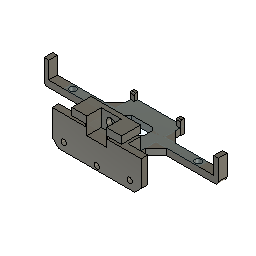
mount v12 (Autodesk Fusion 360 design; units mm, degrees)
Autodesk Fusion 360 part; units mm, degrees
sketch "Sketch1" plane through (0, 0, 0) normal (0, 0, 1) x (1, 0, 0)
  line L0 (51.0982, 3.3166) -> (-51.0982, 3.3166)
  line L1 (-51.0982, 3.3166) -> (-51.0982, -3.3166)
  line L2 (-51.0982, -3.3166) -> (51.0982, -3.3166)
  line L3 (51.0982, -3.3166) -> (51.0982, 3.3166)
  line L4 (51.0982, 3.3166) -> (-51.0982, -3.3166) construction
  line L5 (-51.0982, 3.3166) -> (51.0982, -3.3166) construction
  line L6 (18.7789, 17.5) -> (-18.7789, 17.5)
  line L7 (-18.7789, 17.5) -> (-18.7789, -17.5)
  line L8 (-18.7789, -17.5) -> (18.7789, -17.5)
  line L9 (18.7789, -17.5) -> (18.7789, 17.5)
  line L10 (18.7789, 17.5) -> (-18.7789, -17.5) construction
  line L11 (-18.7789, 17.5) -> (18.7789, -17.5) construction
  dimension "d5" = 35
  constraint horizontal L0
  constraint perpendicular L0 L1
  constraint parallel L0 L2
  constraint parallel L1 L3
  constraint coincident L4 origin
  constraint coincident L5 origin
  constraint horizontal L6
  constraint perpendicular L6 L7
  constraint parallel L6 L8
  constraint parallel L7 L9
  constraint coincident L10 origin
  constraint coincident L11 origin
  measures "d5" distance of L6.start L8.end
extrude "Extrude1" add sketch "Sketch1" along normal blind 5
move_body "Move1" bodies 1 to x (1, 0, 0) y (0, 1, 0) z (0, 0, 1) at (0, 0, -31)
sketch "Sketch2" plane through (0, 0, -31) normal (0, 0, -1) x (1, 0, 0)
  line L0 (18.7789, 3.3166) -> (18.7789, 17.5)
  line L1 (18.7789, 17.5) -> (-18.7789, 17.5)
  line L2 (-18.7789, 17.5) -> (-18.7789, 3.3166)
  line L3 (-18.7789, 3.3166) -> (-51.0982, 3.3166)
  line L4 (-51.0982, 3.3166) -> (-51.0982, -3.3166)
  line L5 (-51.0982, -3.3166) -> (-18.7789, -3.3166)
  line L6 (-18.7789, -3.3166) -> (-18.7789, -17.5)
  line L7 (-18.7789, -17.5) -> (18.7789, -17.5)
  line L8 (18.7789, -17.5) -> (18.7789, -3.3166)
  line L9 (18.7789, -3.3166) -> (51.0982, -3.3166)
  line L10 (51.0982, -3.3166) -> (51.0982, 3.3166)
  line L11 (51.0982, 3.3166) -> (18.7789, 3.3166)
  circle A0 centre (47.5, 0) radius 2.4207
  circle A1 centre (-47.5, 0) radius 2.3964
extrude "Extrude2" cut sketch "Sketch2" against normal blind 5 contours A0 | A1
sketch "Sketch3" plane through (0, 0, -26) normal (0, 0, 1) x (-1, 0, 0)
  circle A0 centre (-47.5, 0) radius 2.4207
  circle A1 centre (47.5, 0) radius 2.3964
  line L0 (-18.7789, 17.5) -> (-18.7789, 3.3166)
  line L1 (-18.7789, 3.3166) -> (-51.0982, 3.3166)
  line L2 (-51.0982, 3.3166) -> (-51.0982, -3.3166)
  line L3 (-51.0982, -3.3166) -> (-18.7789, -3.3166)
  line L4 (-18.7789, -3.3166) -> (-18.7789, -17.5)
  line L5 (-18.7789, -17.5) -> (18.7789, -17.5)
  line L6 (18.7789, -17.5) -> (18.7789, -3.3166)
  line L7 (18.7789, -3.3166) -> (51.0982, -3.3166)
  line L8 (51.0982, -3.3166) -> (51.0982, 3.3166)
  line L9 (51.0982, 3.3166) -> (18.7789, 3.3166)
  line L10 (18.7789, 3.3166) -> (18.7789, 17.5)
  line L11 (18.7789, 17.5) -> (-18.7789, 17.5)
extrude "Extrude3" add 1 faces at (-6.2596, -17.5, -27.6667) along direction (0, -1, 0) blind 12
sketch "Sketch4" plane through (0, 0, -26) normal (0, 0, 1) x (-1, 0, 0)
  circle A0 centre (-47.5, 0) radius 2.4207
  circle A1 centre (47.5, 0) radius 2.3964
  line L0 (-18.7789, 29.5) -> (-18.7789, 3.3166)
  line L1 (-18.7789, 3.3166) -> (-51.0982, 3.3166)
  line L2 (-51.0982, 3.3166) -> (-51.0982, -3.3166)
  line L3 (-51.0982, -3.3166) -> (-18.7789, -3.3166)
  line L4 (-18.7789, -3.3166) -> (-18.7789, -17.5)
  line L5 (-18.7789, -17.5) -> (18.7789, -17.5)
  line L6 (18.7789, -17.5) -> (18.7789, -3.3166)
  line L7 (18.7789, -3.3166) -> (51.0982, -3.3166)
  line L8 (51.0982, -3.3166) -> (51.0982, 3.3166)
  line L9 (51.0982, 3.3166) -> (18.7789, 3.3166)
  line L10 (18.7789, 3.3166) -> (18.7789, 29.5)
  line L11 (18.7789, 29.5) -> (-18.7789, 29.5)
  line L12 (18.7789, 29.5) -> (-18.7789, 29.5)
  line L13 (-18.7789, 29.5) -> (-18.7789, 15.0044)
  line L14 (-18.7789, 15.0044) -> (18.7789, 15.0044)
  line L15 (18.7789, 15.0044) -> (18.7789, 29.5)
  constraint horizontal L12
  constraint vertical L13
  constraint horizontal L14
  constraint vertical L15
  constraint coincident L0 L13.end
  constraint coincident L10.end L11.start
extrude "Extrude4" add sketch "Sketch4" along normal blind 17 contours L0 L10 L11 L12 L13 L14 L15
sketch "Sketch5" plane through (0, -29.5, 0) normal (0, -1, 0) x (1, 0, 0)
  line L0 (-18.7789, -31) -> (18.7789, -31)
  line L1 (18.7789, -31) -> (18.7789, -9)
  line L2 (18.7789, -9) -> (-18.7789, -9)
  line L3 (-18.7789, -9) -> (-18.7789, -31)
  line L4 (-7.4893, -9) -> (7.5, -9)
  line L5 (7.5, -9) -> (7.5, -22)
  line L6 (7.5, -22) -> (-7.4893, -22)
  line L7 (-7.4893, -22) -> (-7.4893, -9)
  constraint horizontal L4
  constraint vertical L5
  constraint horizontal L6
  constraint vertical L7
  constraint coincident L2 L4.start
extrude "Extrude5" cut sketch "Sketch5" against normal blind 11 contours L2 L4 L5 L6 L7
sketch "Sketch6" plane through (0, -29.5, 0) normal (0, -1, 0) x (1, 0, 0)
  line L0 (-7.4893, -22) -> (-7.4893, -9)
  line L1 (-7.4893, -9) -> (-18.7789, -9)
  line L2 (-18.7789, -9) -> (-18.7789, -31)
  line L3 (-18.7789, -31) -> (18.7789, -31)
  line L4 (18.7789, -31) -> (18.7789, -9)
  line L5 (18.7789, -9) -> (7.5, -9)
  line L6 (7.5, -9) -> (7.5, -22)
  line L7 (7.5, -22) -> (-7.4893, -22)
  line L8 (-18.7789, -14.4743) -> (-8.5, -14.4743)
  line L9 (-8.5, -14.4743) -> (-8.5, -16.5)
  line L10 (-8.5, -16.5) -> (-18.7789, -16.5)
  line L11 (-18.7789, -16.5) -> (-18.7789, -14.4743)
  line L12 (18.7789, -14.4808) -> (8.5, -14.4808)
  line L13 (8.5, -14.4808) -> (8.5, -16.5)
  line L14 (8.5, -16.5) -> (18.7789, -16.5)
  line L15 (18.7789, -16.5) -> (18.7789, -14.4808)
  constraint horizontal L8
  constraint vertical L9
  constraint horizontal L10
  constraint vertical L11
  constraint coincident L2 L8.start
  constraint horizontal L12
  constraint vertical L13
  constraint horizontal L14
  constraint vertical L15
  constraint coincident L4 L12.start
extrude "Extrude6" cut sketch "Sketch6" against normal blind 18 contours L2 L8 L9 L10 L11 | L4 L12 L13 L14 L15
sketch "Sketch7" plane through (-18.7789, 0, 0) normal (-1, 0, 0) x (0, -1, 0)
  line L0 (29.5, -16.5) -> (15.0044, -16.5)
  line L1 (15.0044, -16.5) -> (15.0044, -26)
  line L2 (15.0044, -26) -> (3.3166, -26)
  line L3 (3.3166, -26) -> (3.3166, -31)
  line L4 (3.3166, -31) -> (29.5, -31)
  line L5 (29.5, -31) -> (29.5, -16.5)
  line L6 (29.5, -31) -> (24.5, -31)
  line L7 (24.5, -31) -> (24.5, -16.5)
  line L8 (24.5, -16.5) -> (29.5, -16.5)
  line L9 (29.5, -16.5) -> (29.5, -31)
  dimension "d14" = 5
  constraint horizontal L6
  constraint vertical L7
  constraint horizontal L8
  constraint vertical L9
  constraint coincident L4.end L5.start
  measures "d14" distance of L4.end L6.end
sketch "Sketch8" plane through (18.7789, 0, 0) normal (1, 0, 0) x (0, 1, 0)
  line L0 (-15.0044, -16.5) -> (-29.5, -16.5)
  line L1 (-29.5, -16.5) -> (-29.5, -31)
  line L2 (-29.5, -31) -> (-3.3166, -31)
  line L3 (-3.3166, -31) -> (-3.3166, -26)
  line L4 (-3.3166, -26) -> (-15.0044, -26)
  line L5 (-15.0044, -26) -> (-15.0044, -16.5)
  line L6 (-29.5, -31) -> (-24.5, -31)
  line L7 (-24.5, -31) -> (-24.5, -16.5)
  line L8 (-24.5, -16.5) -> (-29.5, -16.5)
  line L9 (-29.5, -16.5) -> (-29.5, -31)
  dimension "d15" = 5
  constraint horizontal L6
  constraint vertical L7
  constraint horizontal L8
  constraint vertical L9
  constraint coincident L1.end L2.start
  measures "d15" distance of L1.end L6.end
extrude "Extrude7" add sketch "Sketch7" along normal blind 15 contours L0 L4 L5 L6 L7 L8 L9
extrude "Extrude8" add sketch "Sketch8" along normal blind 15 contours L0 L1 L2 L6 L7 L8 L9
sketch "Sketch9" plane through (0, 0, -31) normal (0, 0, -1) x (1, 0, 0)
  circle A0 centre (47.5, 0) radius 2.4207
  circle A1 centre (-47.5, 0) radius 2.3964
  line L0 (33.7789, 29.5) -> (-33.7789, 29.5)
  line L1 (-33.7789, 29.5) -> (-33.7789, 24.5)
  line L2 (-33.7789, 24.5) -> (-18.7789, 24.5)
  line L3 (-18.7789, 24.5) -> (-18.7789, 3.3166)
  line L4 (-18.7789, 3.3166) -> (-51.0982, 3.3166)
  line L5 (-51.0982, 3.3166) -> (-51.0982, -3.3166)
  line L6 (-51.0982, -3.3166) -> (-18.7789, -3.3166)
  line L7 (-18.7789, -3.3166) -> (-18.7789, -17.5)
  line L8 (-18.7789, -17.5) -> (18.7789, -17.5)
  line L9 (18.7789, -17.5) -> (18.7789, -3.3166)
  line L10 (18.7789, -3.3166) -> (51.0982, -3.3166)
  line L11 (51.0982, -3.3166) -> (51.0982, 3.3166)
  line L12 (51.0982, 3.3166) -> (18.7789, 3.3166)
  line L13 (18.7789, 3.3166) -> (18.7789, 24.5)
  line L14 (18.7789, 24.5) -> (33.7789, 24.5)
  line L15 (33.7789, 24.5) -> (33.7789, 29.5)
  line L16 (33.7789, 29.5) -> (-33.7789, 29.5)
  line L17 (-33.7789, 29.5) -> (-33.7789, 24.5)
  line L18 (-33.7789, 24.5) -> (33.7789, 24.5)
  line L19 (33.7789, 24.5) -> (33.7789, 29.5)
  constraint horizontal L16
  constraint vertical L17
  constraint horizontal L18
  constraint vertical L19
  constraint coincident L1.end L2.start
  constraint coincident L0.start L15.end
extrude "Extrude9" add sketch "Sketch9" along normal blind 10 contours L0 L1 L2 L14 L15 L16 L17 L18 L19
chamfer "Chamfer1" distance 5 angle 45 1 edges at (33.7789, -27, -41)
chamfer "Chamfer2" distance 5 angle 45 1 edges at (-33.7789, -27, -41)
sketch "Sketch10" plane through (0, 0, -31) normal (0, 0, -1) x (1, 0, 0)
  line L0 (18.7789, 24.5) -> (-18.7789, 24.5)
  line L1 (-18.7789, 24.5) -> (-18.7789, 3.3166)
  line L2 (-18.7789, 3.3166) -> (-51.0982, 3.3166)
  line L3 (-51.0982, 3.3166) -> (-51.0982, -3.3166)
  line L4 (-51.0982, -3.3166) -> (-18.7789, -3.3166)
  line L5 (-18.7789, -3.3166) -> (-18.7789, -17.5)
  line L6 (-18.7789, -17.5) -> (18.7789, -17.5)
  line L7 (18.7789, -17.5) -> (18.7789, -3.3166)
  line L8 (18.7789, -3.3166) -> (51.0982, -3.3166)
  line L9 (51.0982, -3.3166) -> (51.0982, 3.3166)
  line L10 (51.0982, 3.3166) -> (18.7789, 3.3166)
  line L11 (18.7789, 3.3166) -> (18.7789, 24.5)
  circle A0 centre (47.5, 0) radius 2.4207
  circle A1 centre (-47.5, 0) radius 2.3964
  line L12 (18.7789, 24.5) -> (16.7789, 24.5)
  line L13 (16.7789, 24.5) -> (16.7789, 20)
  line L14 (16.7789, 20) -> (18.7789, 20)
  line L15 (18.7789, 20) -> (18.7789, 24.5)
  line L16 (13.7789, 20) -> (11.7789, 20)
  line L17 (11.7789, 20) -> (11.7789, 24.5)
  line L18 (11.7789, 24.5) -> (13.7789, 24.5)
  line L19 (13.7789, 24.5) -> (13.7789, 20)
  line L20 (-18.7789, 24.5) -> (-16.7789, 24.5)
  line L21 (-16.7789, 24.5) -> (-16.7789, 20)
  line L22 (-16.7789, 20) -> (-18.7789, 20)
  line L23 (-18.7789, 20) -> (-18.7789, 24.5)
  line L24 (-13.7789, 24.5) -> (-11.7789, 24.5)
  line L25 (-11.7789, 24.5) -> (-11.7789, 20)
  line L26 (-11.7789, 20) -> (-13.7789, 20)
  line L27 (-13.7789, 20) -> (-13.7789, 24.5)
  line L28 (8.7789, 24.5) -> (6.7789, 24.5)
  line L29 (6.7789, 24.5) -> (6.7789, 20)
  line L30 (6.7789, 20) -> (8.7789, 20)
  line L31 (8.7789, 20) -> (8.7789, 24.5)
  line L32 (-8.7789, 24.5) -> (-6.7789, 24.5)
  line L33 (-6.7789, 24.5) -> (-6.7789, 20)
  line L34 (-6.7789, 20) -> (-8.7789, 20)
  line L35 (-8.7789, 20) -> (-8.7789, 24.5)
  line L36 (1.5061, 24.5) -> (-1.5049, 24.5)
  line L37 (-1.5049, 24.5) -> (-1.5049, 20)
  line L38 (-1.5049, 20) -> (1.5061, 20)
  line L39 (1.5061, 20) -> (1.5061, 24.5)
  dimension "d24" = 2
  dimension "d25" = 4.5
  dimension "d26" = 3
  dimension "d27" = 2
  dimension "d28" = 4.5
  dimension "d29" = 4.5
  dimension "d30" = 2
  dimension "d31" = 3
  dimension "d32" = 4.5
  dimension "d33" = 2
  dimension "d34" = 2
  dimension "d35" = 3
  dimension "d36" = 4.5
  dimension "d37" = 3
  dimension "d38" = 4.5
  dimension "d39" = 2
  dimension "d40" = 5.2728
  dimension "d41" = 5.274
  dimension "d42" = 3.0111
  constraint horizontal L12
  constraint vertical L13
  constraint horizontal L14
  constraint vertical L15
  constraint coincident L0.start L11.end
  constraint horizontal L16
  constraint vertical L17
  constraint horizontal L18
  constraint vertical L19
  constraint coincident L0 L17.end
  constraint horizontal L20
  constraint vertical L21
  constraint horizontal L22
  constraint vertical L23
  constraint coincident L0.end L1.start
  constraint horizontal L24
  constraint vertical L25
  constraint horizontal L26
  constraint vertical L27
  constraint coincident L0 L24.start
  constraint horizontal L28
  constraint vertical L29
  constraint horizontal L30
  constraint vertical L31
  constraint coincident L0 L28.start
  constraint horizontal L32
  constraint vertical L33
  constraint horizontal L34
  constraint vertical L35
  constraint coincident L0 L32.start
  constraint horizontal L36
  constraint vertical L37
  constraint horizontal L38
  constraint vertical L39
  constraint coincident L0 L36.start
  measures "d24" distance of L0.start L12.end
  measures "d25" distance of L12.end L13.end
  measures "d26" distance of L13.end L16.start
  measures "d27" distance of L17.end L18.end
  measures "d28" distance of L16.end L17.end
  measures "d29" distance of L0.end L22.end
  measures "d30" distance of L21.end L22.end
  measures "d31" distance of L21.end L26.end
  measures "d32" distance of L24.start L26.end
  measures "d33" distance of L24.start L24.end
  measures "d34" distance of L29.end L30.end
  measures "d35" horizontal distance of L16.end L30.end
  measures "d36" distance of L28.end L29.end
  measures "d37" distance of L25.end L34.end
  measures "d38" distance of L32.start L34.end
  measures "d39" distance of L32.start L32.end
  measures "d40" distance of L29.end L38.end
  measures "d41" distance of L33.end L37.end
  measures "d42" distance of L37.end L38.end
extrude "Extrude10" add sketch "Sketch10" along normal blind 3 contours L0 L11 L12 L13 L14 L15 | L0 L16 L17 L18 L19 | L0 L28 L29 L30 L31 | L0 L36 L37 L38 L39 | L0 L32 L33 L34 L35 | L0 L24 L25 L26 L27 | L0 L1 L20 L21 L22 L23
chamfer "Chamfer3" distance 2.5 angle 45 7 edges at (-17.7789, -20, -34) (-12.7789, -20, -34) (-7.7789, -20, -34) (0.0006, -20, -34) (7.7789, -20, -34) (12.7789, -20, -34) (17.7789, -20, -34)
sketch "Sketch11" plane through (0, -24.5, 0) normal (0, 1, 0) x (-1, 0, 0)
  line L0 (16.7789, -34) -> (16.7789, -31)
  line L1 (16.7789, -31) -> (13.7789, -31)
  line L2 (13.7789, -31) -> (13.7789, -34)
  line L3 (13.7789, -34) -> (11.7789, -34)
  line L4 (11.7789, -34) -> (11.7789, -31)
  line L5 (11.7789, -31) -> (8.7789, -31)
  line L6 (8.7789, -31) -> (8.7789, -34)
  line L7 (8.7789, -34) -> (6.7789, -34)
  line L8 (6.7789, -34) -> (6.7789, -31)
  line L9 (6.7789, -31) -> (1.5049, -31)
  line L10 (1.5049, -31) -> (1.5049, -34)
  line L11 (1.5049, -34) -> (-1.5061, -34)
  line L12 (-1.5061, -34) -> (-1.5061, -31)
  line L13 (-1.5061, -31) -> (-6.7789, -31)
  line L14 (-6.7789, -31) -> (-6.7789, -34)
  line L15 (-6.7789, -34) -> (-8.7789, -34)
  line L16 (-8.7789, -34) -> (-8.7789, -31)
  line L17 (-8.7789, -31) -> (-11.7789, -31)
  line L18 (-11.7789, -31) -> (-11.7789, -34)
  line L19 (-11.7789, -34) -> (-13.7789, -34)
  line L20 (-13.7789, -34) -> (-13.7789, -31)
  line L21 (-13.7789, -31) -> (-16.7789, -31)
  line L22 (-16.7789, -31) -> (-16.7789, -34)
  line L23 (-16.7789, -34) -> (-18.7789, -34)
  line L24 (-18.7789, -34) -> (-18.7789, -16.5)
  line L25 (-18.7789, -16.5) -> (-33.7789, -16.5)
  line L26 (-33.7789, -16.5) -> (-33.7789, -36)
  line L27 (-33.7789, -36) -> (-28.7789, -41)
  line L28 (-28.7789, -41) -> (28.7789, -41)
  line L29 (28.7789, -41) -> (33.7789, -36)
  line L30 (33.7789, -36) -> (33.7789, -16.5)
  line L31 (33.7789, -16.5) -> (18.7789, -16.5)
  line L32 (18.7789, -16.5) -> (18.7789, -34)
  line L33 (18.7789, -34) -> (16.7789, -34)
  circle A0 centre (-25, -35) radius 2
  circle A1 centre (25, -35) radius 2
  circle A2 centre (0, -38) radius 2
  dimension "d46" = 4
  dimension "d47" = 4
  dimension "d48" = 4
  measures "d46" diameter of A0
  measures "d47" diameter of A1
  measures "d48" diameter of A2
extrude "Extrude11" cut sketch "Sketch11" against normal blind 11 contours A0 | A1 | A2
extrude "Extrude12" add 1 faces at (-51.0982, 1.1055, -29.3333) along direction (-1, 0, 0) blind 10
extrude "Extrude13" add 1 faces at (51.0982, -1.1055, -29.3333) along direction (1, 0, 0) blind 10
extrude "Extrude14" add 1 faces at (-61.0982, 1.1055, -29.3333) along direction (-1, 0, 0) blind 5
extrude "Extrude15" add 1 faces at (61.0982, -1.1055, -29.3333) along direction (1, 0, 0) blind 5
sketch "Sketch12" plane through (0, 0, -26) normal (0, 0, 1) x (-1, 0, 0)
  line L0 (18.7789, 15.0044) -> (-18.7789, 15.0044)
  line L1 (-18.7789, 15.0044) -> (-18.7789, 3.3166)
  line L2 (-18.7789, 3.3166) -> (-66.0982, 3.3166)
  line L3 (-66.0982, 3.3166) -> (-66.0982, -3.3166)
  line L4 (-66.0982, -3.3166) -> (-18.7789, -3.3166)
  line L5 (-18.7789, -3.3166) -> (-18.7789, -17.5)
  line L6 (-18.7789, -17.5) -> (18.7789, -17.5)
  line L7 (18.7789, -17.5) -> (18.7789, -3.3166)
  line L8 (18.7789, -3.3166) -> (66.0982, -3.3166)
  line L9 (66.0982, -3.3166) -> (66.0982, 3.3166)
  line L10 (66.0982, 3.3166) -> (18.7789, 3.3166)
  line L11 (18.7789, 3.3166) -> (18.7789, 15.0044)
  circle A0 centre (-47.5, 0) radius 2.4207
  circle A1 centre (47.5, 0) radius 2.3964
  line L12 (66.0982, -3.3166) -> (62.5982, -3.3166)
  line L13 (62.5982, -3.3166) -> (62.5982, 3.3166)
  line L14 (62.5982, 3.3166) -> (66.0982, 3.3166)
  line L15 (66.0982, 3.3166) -> (66.0982, -3.3166)
  line L16 (-66.0982, 3.3166) -> (-62.5982, 3.3166)
  line L17 (-62.5982, 3.3166) -> (-62.5982, -3.3166)
  line L18 (-62.5982, -3.3166) -> (-66.0982, -3.3166)
  line L19 (-66.0982, -3.3166) -> (-66.0982, 3.3166)
  dimension "d59" = 3.5
  dimension "d60" = 3.5
  constraint horizontal L12
  constraint vertical L13
  constraint horizontal L14
  constraint vertical L15
  constraint coincident L8.end L9.start
  constraint horizontal L16
  constraint vertical L17
  constraint horizontal L18
  constraint vertical L19
  constraint coincident L2.end L3.start
  measures "d59" distance of L8.end L12.end
  measures "d60" distance of L2.end L16.end
extrude "Extrude16" add sketch "Sketch12" along normal blind 13 contours L8 L9 L10 L12 L13 L14 L15 | L2 L3 L4 L16 L17 L18 L19
chamfer "Chamfer4" distance 8 angle 45 4 edges at (-18.7789, 3.3166, -28.5) (-18.7789, -3.3166, -28.5) (18.7789, -3.3166, -28.5) (18.7789, 3.3166, -28.5)
sketch "Sketch13" plane through (0, 0, -31) normal (0, 0, -1) x (1, 0, 0)
  line L0 (-16.7789, 24.5) -> (-16.7789, 20)
  line L1 (-16.7789, 20) -> (-18.7789, 20)
  line L2 (-18.7789, 20) -> (-18.7789, 11.3166)
  line L3 (-18.7789, 11.3166) -> (-26.7789, 3.3166)
  line L4 (-26.7789, 3.3166) -> (-66.0982, 3.3166)
  line L5 (-66.0982, 3.3166) -> (-66.0982, -3.3166)
  line L6 (-66.0982, -3.3166) -> (-26.7789, -3.3166)
  line L7 (-26.7789, -3.3166) -> (-18.7789, -11.3166)
  line L8 (-18.7789, -11.3166) -> (-18.7789, -17.5)
  line L9 (-18.7789, -17.5) -> (18.7789, -17.5)
  line L10 (18.7789, -17.5) -> (18.7789, -11.3166)
  line L11 (18.7789, -11.3166) -> (26.7789, -3.3166)
  line L12 (26.7789, -3.3166) -> (66.0982, -3.3166)
  line L13 (66.0982, -3.3166) -> (66.0982, 3.3166)
  line L14 (66.0982, 3.3166) -> (26.7789, 3.3166)
  line L15 (26.7789, 3.3166) -> (18.7789, 11.3166)
  line L16 (18.7789, 11.3166) -> (18.7789, 20)
  line L17 (18.7789, 20) -> (16.7789, 20)
  line L18 (16.7789, 20) -> (16.7789, 24.5)
  line L19 (16.7789, 24.5) -> (13.7789, 24.5)
  line L20 (13.7789, 24.5) -> (13.7789, 20)
  line L21 (13.7789, 20) -> (11.7789, 20)
  line L22 (11.7789, 20) -> (11.7789, 24.5)
  line L23 (11.7789, 24.5) -> (8.7789, 24.5)
  line L24 (8.7789, 24.5) -> (8.7789, 20)
  line L25 (8.7789, 20) -> (6.7789, 20)
  line L26 (6.7789, 20) -> (6.7789, 24.5)
  line L27 (6.7789, 24.5) -> (1.5061, 24.5)
  line L28 (1.5061, 24.5) -> (1.5061, 20)
  line L29 (1.5061, 20) -> (-1.5049, 20)
  line L30 (-1.5049, 20) -> (-1.5049, 24.5)
  line L31 (-1.5049, 24.5) -> (-6.7789, 24.5)
  line L32 (-6.7789, 24.5) -> (-6.7789, 20)
  line L33 (-6.7789, 20) -> (-8.7789, 20)
  line L34 (-8.7789, 20) -> (-8.7789, 24.5)
  line L35 (-8.7789, 24.5) -> (-11.7789, 24.5)
  line L36 (-11.7789, 24.5) -> (-11.7789, 20)
  line L37 (-11.7789, 20) -> (-13.7789, 20)
  line L38 (-13.7789, 20) -> (-13.7789, 24.5)
  line L39 (-13.7789, 24.5) -> (-16.7789, 24.5)
  circle A0 centre (-47.5, 0) radius 2.3964
  circle A1 centre (47.5, 0) radius 2.4207
  line L40 (10, 5) -> (-10, 5)
  line L41 (-10, 5) -> (-10, -5)
  line L42 (-10, -5) -> (10, -5)
  line L43 (10, -5) -> (10, 5)
  line L44 (10, 5) -> (-10, -5) construction
  line L45 (-10, 5) -> (10, -5) construction
  dimension "d64" = 20
  dimension "d65" = 10
  constraint horizontal L40
  constraint perpendicular L40 L41
  constraint parallel L40 L42
  constraint parallel L41 L43
  constraint coincident L44 origin
  constraint coincident L45 origin
  measures "d64" distance of L41.end L42.end
  measures "d65" distance of L40.end L41.end
extrude "Extrude17" cut sketch "Sketch13" against normal blind 22 contours L40 L41 L42 L43
chamfer "Chamfer5" distance 2 angle 45 4 edges at (10, -5, -28.5) (10, 5, -28.5) (-10, 5, -28.5) (-10, -5, -28.5)
fillet "Fillet1" radius 2.5 2 edges at (66.0982, 0, -31) (-66.0982, 0, -31)
sketch "Sketch14" plane through (0, -18.5, 0) normal (0, -1, 0) x (1, 0, 0)
  line L0 (-7.4893, -22) -> (7.5, -22)
  line L1 (7.5, -22) -> (7.5, -9)
  line L2 (7.5, -9) -> (-7.4893, -9)
  line L3 (-7.4893, -9) -> (-7.4893, -22)
  circle A0 centre (0, -15.8) radius 3.6878
extrude "Extrude18" cut sketch "Sketch14" against normal blind 7 contours A0
sketch "Sketch15" plane through (-18.7789, 0, 0) normal (-1, 0, 0) x (0, -1, 0)
  line L0 (11.3166, -26) -> (11.3166, -31)
  line L1 (11.3166, -31) -> (20, -31)
  line L2 (20, -31) -> (20, -31.5)
  line L3 (20, -31.5) -> (22.5, -34)
  line L4 (22.5, -34) -> (24.5, -34)
  line L5 (24.5, -34) -> (24.5, -16.5)
  line L6 (24.5, -16.5) -> (15.0044, -16.5)
  line L7 (15.0044, -16.5) -> (15.0044, -26)
  line L8 (15.0044, -26) -> (11.3166, -26)
  line L9 (20, -25) -> (24.5, -25)
  line L10 (24.5, -25) -> (24.5, -20.5)
  line L11 (24.5, -20.5) -> (20, -20.5)
  line L12 (20, -20.5) -> (20, -25)
  dimension "d73" = 4.5
  constraint horizontal L9
  constraint vertical L10
  constraint horizontal L11
  constraint vertical L12
  measures "d73" distance of L9.start L11.end
sketch "Sketch16" plane through (18.7789, 0, 0) normal (1, 0, 0) x (0, 1, 0)
  line L0 (-11.3166, -31) -> (-11.3166, -26)
  line L1 (-11.3166, -26) -> (-15.0044, -26)
  line L2 (-15.0044, -26) -> (-15.0044, -16.5)
  line L3 (-15.0044, -16.5) -> (-24.5, -16.5)
  line L4 (-24.5, -16.5) -> (-24.5, -34)
  line L5 (-24.5, -34) -> (-22.5, -34)
  line L6 (-22.5, -34) -> (-20, -31.5)
  line L7 (-20, -31.5) -> (-20, -31)
  line L8 (-20, -31) -> (-11.3166, -31)
  line L9 (-24.5, -24.9845) -> (-20, -24.9845)
  line L10 (-20, -24.9845) -> (-20, -20.5)
  line L11 (-20, -20.5) -> (-24.5, -20.5)
  line L12 (-24.5, -20.5) -> (-24.5, -24.9845)
  constraint horizontal L9
  constraint vertical L10
  constraint horizontal L11
  constraint vertical L12
  constraint coincident L4 L9.start
extrude "Extrude19" add sketch "Sketch15" along normal blind 4.5 contours L5 L9 L10 L11 L12
extrude "Extrude20" add sketch "Sketch16" along normal blind 4.5 contours L4 L9 L10 L11 L12
chamfer "Chamfer6" distance 4.5 angle 45 2 edges at (23.2789, -20, -22.7423) (-23.2789, -20, -22.75)
fillet "Fillet2" radius 1 7 edges at (17.7789, -22.5, -34) (12.7789, -22.5, -34) (7.7789, -22.5, -34) (0.0006, -22.5, -34) (-7.7789, -22.5, -34) (-12.7789, -22.5, -34) (-17.7789, -22.5, -34)
sketch "Sketch17" plane through (0, 0, -26) normal (0, 0, 1) x (1, 0, 0)
  line L0 (-16, 15) -> (-19, 15)
  line L1 (-19, 15) -> (-19, 18)
  line L2 (-19, 18) -> (-16, 18)
  line L3 (-16, 18) -> (-16, 15)
  line L4 (16, 15) -> (19, 15)
  line L5 (19, 15) -> (19, 18)
  line L6 (19, 18) -> (16, 18)
  line L7 (16, 18) -> (16, 15)
  constraint horizontal L0
  constraint vertical L1
  constraint horizontal L2
  constraint vertical L3
  constraint horizontal L4
  constraint vertical L5
  constraint horizontal L6
  constraint vertical L7
extrude "Extrude21" add sketch "Sketch17" along normal blind 5
move_face "OffsetFaces1" offset 5 2 faces at (-17.9263, 17.8333, -26) (17.9263, 17.8333, -26)
fillet "Fillet3" radius 1 2 edges at (-17.5, 15, -21) (17.5, 15, -21)
fillet "Fillet4" radius 0.5 2 edges at (16, 18, -26) (-16, 18, -26)
delete_face "DeleteFace1" 1 faces at (-1.5049, -22.2357, -32.069)
move_face "OffsetFaces2" offset 8 1 faces at (16.7789, -22.2357, -32.069)
extrude "Extrude22" cut 1 faces at (-8.7789, -22.2357, -32.069) along direction (-1, 0, 0) blind 8
move_face "OffsetFaces3" offset 8 1 faces at (-8.7789, -22.2357, -32.069)
